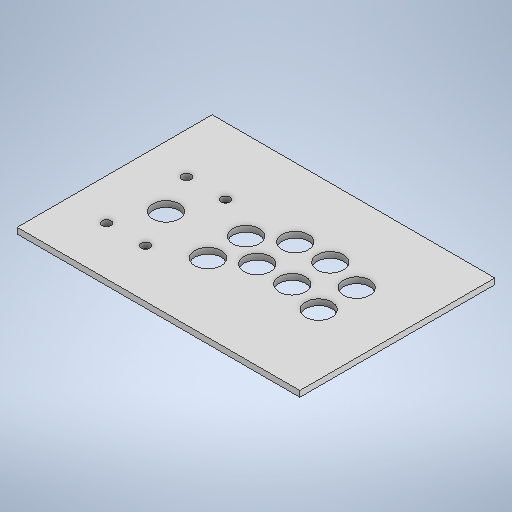
# Autodesk Inventor part: sega_straight_b2_v1
Saved by Autodesk Inventor 2025 (Build 290162010, 162A)
## iProperties
Created: 2022-12-25
Part Number: sega_straight_b2_v1
Material: Generic
Document SubType Name: Modeling
Designer: Bunny
Density: 1 g/cm^3
Appearance: Default
Author: Bunny
Autodesk Inventor part; units mm, degrees
ref_plane "YZ Plane" through (0, 0, 0) normal (1, 0, 0) x (0, 1, 0)
ref_plane "XZ Plane" through (0, 0, 0) normal (0, 1, 0) x (-1, 0, 0)
ref_plane "XY Plane" through (0, 0, 0) normal (0, 0, 1) x (1, 0, 0)
sketch "Sketch1" plane through (0, 0, 0) normal (0, 1, 0) x (-1, 0, 0)
  line L0 (145, -100) -> (-145, -100)
  line L1 (-145, -100) -> (-145, 100)
  line L2 (-145, 100) -> (145, 100)
  line L3 (145, 100) -> (145, -100)
  line L4 (210, 0) -> (-210, 0) projected
  line L5 (0, -140) -> (0, 140) projected
  point P0 (0, 0)
  dimension "d30" = 290
  dimension "d31" = 200
  constraints: 8 end point, 2 parallel, 1 horizontal, 1 perpendicular, 2 other
  measures "d30" distance of L0.start L0.end
  measures "d31" distance of L0.end L1.end
extrude "Extrusion1" add sketch "Sketch1" along normal blind 6
sketch "Sketch2" plane through (0, 6, 0) normal (0, 1, 0) x (1, 0, 0)
  circle A0 centre (-19.75, -29.5) radius 13.5
  circle A1 centre (-82.75, -9.5) radius 13.5
  circle A2 centre (-19.75, 9.5) radius 13.5
  circle A3 centre (46.75, 29.5) radius 13.5
  circle A4 centre (82.75, 20.5) radius 13.5
  circle A5 centre (10.75, 29.5) radius 13.5
  circle A6 centre (10.75, -9.5) radius 13.5
  circle A7 centre (46.75, -9.5) radius 13.5
  circle A8 centre (82.75, -18.5) radius 13.5
  line L0 (-96.25, 43) -> (96.25, 43)
  line L1 (96.25, 43) -> (96.25, -43)
  line L2 (96.25, -43) -> (-96.25, -43)
  line L3 (-96.25, -43) -> (-96.25, 43)
  line L4 (145, 100) -> (-145, 100) projected
  line L5 (145, -100) -> (145, 100) projected
  line L6 (0, 140) -> (0, -140) projected
  line L7 (-210, 0) -> (210, 0) projected
  line L8 (-102.75, 31.5) -> (-62.75, 31.5)
  line L9 (-62.75, 31.5) -> (-62.75, -50.5)
  line L10 (-62.75, -50.5) -> (-102.75, -50.5)
  line L11 (-102.75, -50.5) -> (-102.75, 31.5)
  circle A9 centre (-102.75, 31.5) radius 4.5
  circle A10 centre (-62.75, 31.5) radius 4.5
  circle A11 centre (-102.75, -50.5) radius 4.5
  circle A12 centre (-62.75, -50.5) radius 4.5
  dimension "d3" = 27
  dimension "d19" = 30.5
  dimension "d20" = 36
  dimension "d23" = 19
  dimension "d24" = 9
  dimension "d25" = 36
  dimension "d26" = 11
  dimension "d27" = 9
  dimension "d28" = 11
  dimension "d29" = 63
  dimension "d35" = 41
  dimension "d36" = 41
  dimension "d37" = 20
  dimension "d38" = 20
  dimension "d39" = 9
  dimension "d40" = 9
  dimension "d41" = 9
  dimension "d42" = 9
  constraints: 16 end point, 13 centre point, 8 equal radius, 4 coincident, 4 parallel, 4 tangent, 4 vertical alignment, 3 horizontal alignment, 2 horizontal, 2 perpendicular, 2 other
  measures "d3" diameter of A1
  measures "d19" horizontal distance of A0.centre A6.centre
  measures "d20" distance of A7.centre A6.centre
  measures "d23" vertical distance of A6.centre A2.centre
  measures "d24" vertical distance of A8.centre A6.centre
  measures "d25" horizontal distance of A8.centre A7.centre
  measures "d26" vertical distance of A0.centre A8.centre
  measures "d27" vertical distance of A4.centre A5.centre
  measures "d28" vertical distance of A2.centre A4.centre
  measures "d29" horizontal distance of A0.centre A1.centre
  measures "d35" distance from line of L8 A1.centre
  measures "d36" distance from line of L10 A1.centre
  measures "d37" distance from line of L11 A1.centre
  measures "d38" distance from line of L9 A1.centre
  measures "d39" diameter of A9
  measures "d40" diameter of A10
  measures "d41" diameter of A11
  measures "d42" diameter of A12
extrude "Extrusion2" cut sketch "Sketch2" against normal blind 30 contours A0 | A8 | L6 A6 L7 | A6 L6 | A12 L10 L9 | L9 L10 A12 | A1 L7 | L7 A1 | L7 A2 | A2 L7 | A10 L8 L9 | L9 L8 A10 | A4 | A3 | A6 L7 | A11 L11 L10 | L10 L11 A11 | L7 A7 | A7 L7 | L6 A5 | A5 L6 | A9 L11 L8 | L8 L11 A9 picked at (6.7806, -6.3333)
equation "\"d30\" = BoxLength"
equation "\"d31\" = BoxWidth"
equation "\"d3\" = JS_Hole_dia"
equation "\"d36\" = 0.5 * JS_SH_L"
equation "\"d37\" = 0.5 * JS_SH_W"
equation "\"d38\" = 0.5 * JS_SH_W"
equation "\"d39\" = JS_SH_top_dia"
equation "\"d40\" = JS_SH_top_dia"
equation "\"d41\" = JS_SH_top_dia"
equation "\"d42\" = JS_SH_top_dia"
equation "\"BoxLength\" = 290"
equation "\"BoxWidth\" = 200"
equation "\"JS_SH_L\" = 82"
equation "\"JS_SH_dia\" = 5"
equation "\"SheetThickness\" = 6"
equation "\"CornerOffset\" = 5"
equation "\"NutS\" = 5.7"
equation "\"NutThreadD2\" = 4.17"
equation "\"SideNutWidth\" = 2.5"
equation "\"JS_Hole_dia\" = 27"
equation "\"JS_SH_top_dia\" = 9"
equation "\"JS_SH_W\" = 40"
body "Solid1"
